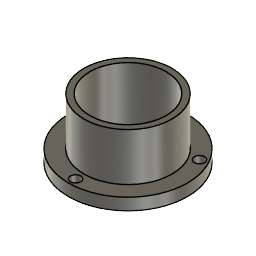
Extractor Prototype (Autodesk Fusion 360 archive; units mm, degrees)
design "ConnectorAttachment"
Autodesk Fusion 360 part; units mm, degrees
sketch "Sketch1" plane through (0, 0, 0) normal (0, 0, 1) x (1, 0, 0)
  circle A0 centre (0, 0) radius 16
  circle A1 centre (0, 0) radius 18.5
  circle A2 centre (0, 0) radius 25
  dimension "d1" = 32
  dimension "d2" = 37
  dimension "d3" = 50
  constraint coincident A0.centre A1.centre
  constraint concentric A0 A1
  measures "d1" diameter of A0
  measures "d2" diameter of A1
  measures "d3" diameter of A2
extrude "Extrude1" add sketch "Sketch1" against normal blind 5 contours A2
extrude "Extrude2" add sketch "Sketch1" against normal blind 5 contours A1
extrude "Extrude3" add sketch "Sketch1" along normal blind 20 contours A1
sketch "Sketch2" plane through (0, 0, 0) normal (0, 0, 1) x (-1, 0, 0)
  circle A0 centre (0, 0) radius 18.5
  circle A1 centre (0, 0) radius 25
  line L0 (0, 0) -> (0, 25) construction
  line L1 (0, 0) -> (-21.6506, -12.5) construction
  line L2 (0, 0) -> (21.6506, -12.5) construction
  circle A2 centre (0, 22) radius 2.15
  circle A3 centre (19.0526, -11) radius 2.15
  circle A4 centre (-19.0526, -11) radius 2.15
  dimension "d10" = 120
  dimension "d11" = 120
  dimension "d12" = 4.3
  dimension "d13" = 22
  dimension "d14" = 4.3
  dimension "d15" = 4.3
  dimension "d16" = 22
  dimension "d17" = 22
  constraint coincident A0.centre A1.centre
  constraint coincident A1 L0.end
  constraint vertical L0
  constraint coincident A1 L1.end
  constraint coincident A1 L2.end
  constraint coincident L0 A2.centre
  constraint coincident L2 A3.centre
  constraint coincident L1 A4.centre
  measures "d10" angle of L0 L2
  measures "d11" angle of L1 L2
  measures "d12" diameter of A2
  measures "d13" distance of A0.centre A2.centre
  measures "d14" diameter of A3
  measures "d15" diameter of A4
  measures "d16" distance of A0.centre A4.centre
  measures "d17" distance of A0.centre A3.centre
extrude "Extrude4" cut sketch "Sketch2" against normal blind 8 contours A2 | A3 | A4

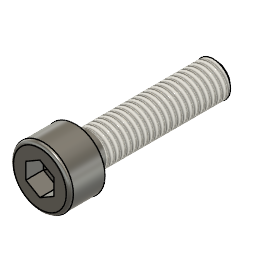
design "Hexagon Socket Head Cap Screw DIN 912 - M5 x 0.8 x 20 Steel 4.6 Plain"
description: Hexagon Socket Head Cap Screw DIN 912 - M5 x 0.8 x 20
part number: DIN 912 - M5 x 0.8 x 20 Steel 4.6 Plain
Autodesk Fusion 360 part; units mm, degrees
sketch "Sketch1" plane through (0, 0, 0) normal (0, 1, 0) x (1, 0, 0)
  line L0 (-2.5, 0) -> (-2.5, 20)
  line L1 (-2.5, 20) -> (0, 20)
  line L2 (0, 20) -> (0, -5)
  line L3 (-2.5, 0) -> (-4.25, 0)
  line L4 (-4.25, 0) -> (-4.25, -5)
  line L5 (-4.25, -5) -> (0, -5)
  dimension "d101" = 20
  dimension "d102" = 5
  dimension "d109" = 8.5
  dimension "d110" = 5
  constraint perpendicular L0 L1
  constraint collinear origin L1.end L2.end
  constraint perpendicular L0 L3
  constraint coincident origin L3
  constraint vertical L2
  constraint coincident L2 L5.end
  constraint perpendicular L2 L5
  measures "d101" distance of origin L1
  measures "d102" distance of L3.end L5
revolve "Revolve1" add sketch "Sketch1" angle 360 about axis through (0, 0, -20) along (0, 0, 1)
ref_plane "WorkPlane1" through (0, 0, 5) normal (0, 0, 1) x (1, 0, 0)
sketch "Sketch6" plane through (0, 0, 5) normal (0, 0, 1) x (1, 0, 0)
  line L0 (0, -2.3094) -> (2, -1.1547)
  line L1 (2, -1.1547) -> (2, 1.1547)
  line L2 (2, 1.1547) -> (0, 2.3094)
  line L3 (0, 2.3094) -> (-2, 1.1547)
  line L4 (-2, 1.1547) -> (-2, -1.1547)
  line L5 (-2, -1.1547) -> (0, -2.3094)
  dimension "d111" = 4
  constraint vertical L1
  measures "d111" distance of L1 L4
extrude "Extrude1" cut sketch "Sketch6" against normal blind 2.5
extrude "Extrude2" cut 1 faces at (-0.6667, -0.3849, 2.5) along direction (0, 0, -1) blind 2.5 draft -85
thread "Thread3" "ISO Metric profile 5.0 M5x0.8 M5x0.8 6g" major diameter 4.901 minor diameter 3.9895 pitch 0.8 angle 60 resizes the face on face at (-2.4969, 0.1246, -13.3333) from (0, 0, -2) to (0, 0, -20)
fillet "Fillet4" radius 0.5 1 edges at (-3.9624, 1.5369, 5)
sketch "Sketch7" plane through (0, 0, 0) normal (0, 1, 0) x (1, 0, 0)
  line L0 (-2.55, 20) -> (-2.55, 19.5092)
  line L1 (-2.55, 19.5092) -> (-2.0092, 20)
  line L2 (0, 20) -> (0, -5)
  line L3 (-2.55, 20) -> (0, 20)
  dimension "d104" = 2.0092
  dimension "d105" = 2.55
  dimension "d106" = 0.4908
  constraint coincident L2.start L3.end
  constraint perpendicular L2 L3
  constraint coincident L1.end L3
  constraint perpendicular L0 L3
  measures "d104" distance of L1.end L2
  measures "d105" distance of L0 L2.start
  measures "d106" distance of L0.end L3
revolve "Revolve3" cut sketch "Sketch7" angle 360 about axis through (0, 0, 1.75) along (0, 0, 1)
equation "adsk_nomlen = 20.00 mm"
equation "adsk_headh = 5.00 mm"
equation "adsk_headdia = 8.50 mm"
equation "adsk_nomdia = 5.00 mm"
equation "adsk_philwidth = 4.00 mm"
equation "d31 = -adsk_phildepth"
equation "adsk_phildepth = 2.50 mm"
equation "d71 = adsk_headh"
equation "d76 = -adsk_phildepth"
equation "adsk_thrlen = 18.00 mm"
equation "d86 = adsk_nomdia * 0.1"
equation "adsk_startlen = 0.49076 mm"
equation "adsk_endpointdia = 4.01848 mm"
equation "d101 = adsk_nomlen"
equation "d102 = adsk_headh"
equation "d104 = adsk_endpointdia / 2"
equation "d105 = adsk_nomdia * 0.51"
equation "d106 = adsk_startlen"
equation "d108 = min(adsk_thrlen; adsk_nomlen - 0.001 mm)"
equation "d109 = adsk_headdia"
equation "d110 = adsk_nomdia"
equation "d111 = adsk_philwidth"

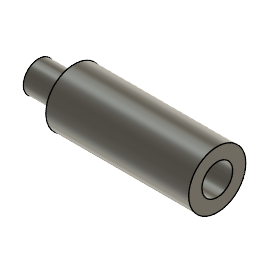
design "4mm OD Threaded Tubing Insert"
Autodesk Fusion 360 part; units mm, degrees
sketch "Sketch1" plane through (0, 0, 0) normal (1, 0, 0) x (0, 1, 0)
  circle A0 centre (0, 0) radius 2.15
  dimension "d1" = 4.3
  constraint coincident A0.centre origin
  measures "d1" diameter of A0
extrude "Extrude1" add sketch "Sketch1" along normal blind 5 makes body 1
sketch "Sketch2" plane through (5, 0, 0) normal (1, 0, 0) x (0, 1, 0)
  circle A0 centre (0, 0) radius 2.15
  circle A1 centre (0, 0) radius 4
  dimension "d4" = 8
  constraint coincident A0.centre A1.centre
  measures "d4" diameter of A1
extrude "Extrude2" add sketch "Sketch2" along normal blind 20 separate body makes body 2

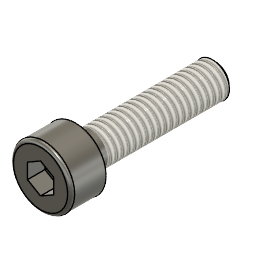
design "Hexagon Socket Head Cap Screw DIN 912 - M4 x 0.7 x 16 Steel 4.6 Plain"
description: Hexagon Socket Head Cap Screw DIN 912 - M4 x 0.7 x 16
part number: DIN 912 - M4 x 0.7 x 16 Steel 4.6 Plain
Autodesk Fusion 360 part; units mm, degrees
sketch "Sketch1" plane through (0, 0, 0) normal (0, 1, 0) x (1, 0, 0)
  line L0 (-2, 0) -> (-2, 16)
  line L1 (-2, 16) -> (0, 16)
  line L2 (0, 16) -> (0, -4)
  line L3 (-2, 0) -> (-3.5, 0)
  line L4 (-3.5, 0) -> (-3.5, -4)
  line L5 (-3.5, -4) -> (0, -4)
  dimension "d101" = 16
  dimension "d102" = 4
  dimension "d109" = 7
  dimension "d110" = 4
  constraint perpendicular L0 L1
  constraint collinear origin L1.end L2.end
  constraint perpendicular L0 L3
  constraint coincident origin L3
  constraint vertical L2
  constraint coincident L2 L5.end
  constraint perpendicular L2 L5
  measures "d101" distance of origin L1
  measures "d102" distance of L3.end L5
revolve "Revolve1" add sketch "Sketch1" angle 360 about axis through (0, 0, -16) along (0, 0, 1)
ref_plane "WorkPlane1" through (0, 0, 4) normal (0, 0, 1) x (1, 0, 0)
sketch "Sketch6" plane through (0, 0, 4) normal (0, 0, 1) x (1, 0, 0)
  line L0 (0, -1.7321) -> (1.5, -0.866)
  line L1 (1.5, -0.866) -> (1.5, 0.866)
  line L2 (1.5, 0.866) -> (0, 1.7321)
  line L3 (0, 1.7321) -> (-1.5, 0.866)
  line L4 (-1.5, 0.866) -> (-1.5, -0.866)
  line L5 (-1.5, -0.866) -> (0, -1.7321)
  dimension "d111" = 3
  constraint vertical L1
  measures "d111" distance of L1 L4
extrude "Extrude1" cut sketch "Sketch6" against normal blind 2
extrude "Extrude2" cut 1 faces at (0.5, 0.2887, 2) along direction (0, 0, -1) blind 2 draft -85
thread "Thread3" "ISO Metric profile 4.0 M4x0.7 M4x0.7 6g" major diameter 3.908 minor diameter 3.111 pitch 0.7 angle 60 resizes the face on face at (-1.9901, 0.1991, -10.6667) from (0, 0, -1.75) to (0, 0, -16)
fillet "Fillet4" radius 0.4 1 edges at (-3.2631, 1.2657, 4)
sketch "Sketch7" plane through (0, 0, 0) normal (0, 1, 0) x (1, 0, 0)
  line L0 (-2.04, 16) -> (-2.04, 15.5706)
  line L1 (-2.04, 15.5706) -> (-1.5706, 16)
  line L2 (0, 16) -> (0, -4)
  line L3 (-2.04, 16) -> (0, 16)
  dimension "d104" = 1.5706
  dimension "d105" = 2.04
  dimension "d106" = 0.4294
  constraint coincident L2.start L3.end
  constraint perpendicular L2 L3
  constraint coincident L1.end L3
  constraint perpendicular L0 L3
  measures "d104" distance of L1.end L2
  measures "d105" distance of L0 L2.start
  measures "d106" distance of L0.end L3
revolve "Revolve3" cut sketch "Sketch7" angle 360 about axis through (0, 0, 1.75) along (0, 0, 1)
equation "adsk_nomlen = 16.00 mm"
equation "adsk_headh = 4.00 mm"
equation "adsk_headdia = 7.00 mm"
equation "adsk_nomdia = 4.00 mm"
equation "adsk_philwidth = 3.00 mm"
equation "d31 = -adsk_phildepth"
equation "adsk_phildepth = 2.00 mm"
equation "d71 = adsk_headh"
equation "d76 = -adsk_phildepth"
equation "adsk_thrlen = 14.25 mm"
equation "d86 = adsk_nomdia * 0.1"
equation "adsk_startlen = 0.429415 mm"
equation "adsk_endpointdia = 3.14117 mm"
equation "d101 = adsk_nomlen"
equation "d102 = adsk_headh"
equation "d104 = adsk_endpointdia / 2"
equation "d105 = adsk_nomdia * 0.51"
equation "d106 = adsk_startlen"
equation "d108 = min(adsk_thrlen; adsk_nomlen - 0.001 mm)"
equation "d109 = adsk_headdia"
equation "d110 = adsk_nomdia"
equation "d111 = adsk_philwidth"
